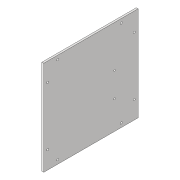
# Autodesk Inventor part: BREEZE-M07
Saved by Autodesk Inventor 2020 (Build 240168000, 168)
## iProperties
Created: 2020-04-12
Part Number: BREEZE-M07
Material: Generic
Description: SIDE PANEL
Document SubType Name: Modeling
Designer: John K
Density: 1 g/cm^3
Appearance: Default
Author: John K
Autodesk Inventor part; units mm, degrees
ref_plane "YZ Plane" through (0, 0, 0) normal (1, 0, 0) x (0, 1, 0)
ref_plane "XZ Plane" through (0, 0, 0) normal (0, 1, 0) x (-1, 0, 0)
ref_plane "XY Plane" through (0, 0, 0) normal (0, 0, 1) x (1, 0, 0)
sketch "Face" plane through (0, 0, 0) normal (0, 0, 1) x (1, 0, 0)
  circle A0 centre (230.4851, 204.87) radius 2.6
  circle A1 centre (45, 10) radius 2.6
  circle A2 centre (193.5381, 10) radius 2.6
  circle A3 centre (10, 204.87) radius 2.6
  circle A4 centre (193.5381, 230.5) radius 2.6
  circle A5 centre (10, 42.67) radius 2.6
  circle A6 centre (230.4851, 42.67) radius 2.6
  circle A7 centre (45, 230.5) radius 2.6
  line L0 (240.4851, 0) -> (0, 0)
  line L1 (240.4851, 0) -> (240.4851, 240.5)
  line L2 (0, 240.5) -> (240.4851, 240.5)
  line L3 (0, 240.5) -> (0, 0)
  point P0 (115.8277, 117.0745)
  point P1 (0, 0)
sketch "Sketch1" plane through (0, 0, 0) normal (1, 0, 0) x (0, 1, 0)
  circle A0 centre (110.2425, 84.62) radius 2.6
  circle A1 centre (-75.2425, -110.25) radius 2.6
  circle A2 centre (73.2955, -110.25) radius 2.6
  circle A3 centre (-110.2425, 84.62) radius 2.6
  circle A4 centre (73.2955, 110.25) radius 2.6
  circle A5 centre (-110.2425, -77.58) radius 2.6
  circle A6 centre (110.2425, -77.58) radius 2.6
  circle A7 centre (-75.2425, 110.25) radius 2.6
  line L0 (120.2425, -120.25) -> (-120.2425, -120.25)
  line L1 (120.2425, -120.25) -> (120.2425, 120.25)
  line L2 (-120.2425, 120.25) -> (120.2425, 120.25)
  line L3 (-120.2425, 120.25) -> (-120.2425, -120.25)
  point P0 (0, 0)
  point P1 (-120.2425, 0)
  point P2 (0, 120.25)
  constraints: 1 horizontal alignment, 1 vertical alignment, 2 other
extrude "Extrusion1" add sketch "Sketch1" along normal mid plane 4.75
sketch "Sketch2" plane through (-2.375, 0, 0) normal (-1, 0, 0) x (0, 0, 1)
  arc A0 (-55.5931, 11.2793) -> (-64.9069, 11.2793) centre (-60.25, 14.31) ccw projected
  arc A1 (-64.9069, -45.3655) -> (-55.5931, -45.3655) centre (-60.25, -48.3962) ccw projected
hole "Hole1" at (-2.375, 14.31, -60.25) at (-2.375, -48.3962, -60.25) direction (1, 0, 0) diameter 4.5 end through all clearance for "Socket Head Cap Screw" size "M4" standard "Ansi Metric M Profile"
body "Solid1"
